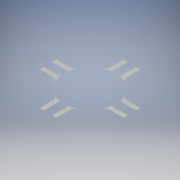
# Autodesk Inventor part: center
Saved by Autodesk Inventor 2016 (Build 200138000, 138)
## iProperties
Created: 2016-02-28
Part Number: center
Material: Generic
Document SubType Name: Modeling
Designer: Matt Ruffner
Density: 1 g/cm^3
Appearance: Default
Author: Matt Ruffner
Autodesk Inventor part; units mm, degrees
ref_plane "YZ Plane" through (0, 0, 0) normal (1, 0, 0) x (0, 1, 0)
ref_plane "XZ Plane" through (0, 0, 0) normal (0, 1, 0) x (-1, 0, 0)
ref_plane "XY Plane" through (0, 0, 0) normal (0, 0, 1) x (1, 0, 0)
sketch "Sketch1" plane through (0, 0, 0) normal (0, 1, 0) x (-1, 0, 0)
  circle A0 centre (0, 0) radius 4.318
  line L0 (0, -31.496) -> (5.08, -31.496)
  line L1 (0, -31.496) -> (-5.08, -31.496)
  line L2 (31.496, 0) -> (31.496, 5.08)
  line L3 (31.496, 0) -> (31.496, -5.08)
  line L4 (0, 31.496) -> (-5.08, 31.496)
  line L5 (0, 31.496) -> (5.08, 31.496)
  line L6 (-31.496, 0) -> (-31.496, -5.08)
  line L7 (-31.496, 0) -> (-31.496, 5.08)
  line L8 (31.496, 5.08) -> (50.5454, 5.08)
  line L9 (31.496, -5.08) -> (50.5454, -5.08)
  line L10 (5.08, -31.496) -> (5.08, -50.5454)
  line L11 (-5.08, -31.496) -> (-5.08, -50.5454)
  line L12 (-31.496, -5.08) -> (-50.5454, -5.08)
  line L13 (-31.496, 5.08) -> (-50.5454, 5.08)
  line L14 (-5.08, 31.496) -> (-5.08, 50.5454)
  line L15 (5.08, 31.496) -> (5.08, 50.5454)
  line L16 (-50.5454, 5.08) -> (-50.5454, 10.16)
  line L17 (-50.5454, -5.08) -> (-50.5454, -10.16)
  line L18 (-5.08, -50.5454) -> (-10.16, -50.5454)
  line L19 (5.08, -50.5454) -> (10.16, -50.5454)
  line L20 (50.5454, -5.08) -> (50.5454, -10.16)
  line L21 (50.5454, 5.08) -> (50.5454, 10.16)
  line L22 (5.08, 50.5454) -> (10.16, 50.5454)
  line L23 (-5.08, 50.5454) -> (-10.16, 50.5454)
  line L24 (-10.16, 50.5454) -> (-10.16, 29.8123)
  line L25 (10.16, 50.5454) -> (10.16, 29.8123)
  line L26 (-50.5454, 10.16) -> (-29.8123, 10.16)
  line L27 (-50.5454, -10.16) -> (-29.8123, -10.16)
  line L28 (-10.16, -50.5454) -> (-10.16, -29.8123)
  line L29 (10.16, -50.5454) -> (10.16, -29.8123)
  line L30 (50.5454, -10.16) -> (29.8123, -10.16)
  line L31 (50.5454, 10.16) -> (29.8123, 10.16)
  arc A1 (-10.16, 29.8123) -> (-29.8123, 10.16) centre (0, 0) ccw
  arc A2 (-29.8123, -10.16) -> (-10.16, -29.8123) centre (0, 0) ccw
  arc A3 (10.16, -29.8123) -> (29.8123, -10.16) centre (0, 0) ccw
  arc A4 (29.8123, 10.16) -> (10.16, 29.8123) centre (0, 0) ccw
  dimension "d7" = 360
  dimension "d13" = 360
  dimension "d0" = 8.636
  dimension "d9" = 5.08
  dimension "d10" = 5.08
  constraints: 64 end point, 8 horizontal, 8 point on circle, 5 centre point, 4 parallel, 4 vertical, 3 perpendicular, 1 coincident, 1 point on line, 46 other
  measures "d0" diameter of A0
  measures "d9" distance of L13.end L16.end
  measures "d10" distance of L12.end L17.end
extrude "Extrusion1" add sketch "Sketch1" along normal blind 7.62
sketch "Sketch2" plane through (10.16, 0, 50.5454) normal (1, 0, 0) x (0, 0, -1)
  line L0 (0, 0) -> (20.7331, 0) projected
  circle A0 centre (11.1754, 3.81) radius 1.651
  point P0 (50.5454, 0)
  dimension "d19" = 3.302
  constraints: 1 centre point
  measures "d19" diameter of A0
extrude "Extrusion2" cut sketch "Sketch2" against normal up to surface (20.32 mm away)
pattern_circular "Circular Pattern1" count 4 over 360 about axis through (0, 0, 0) along (0, 1, 0) of "Extrusion2"
sketch "Sketch3" plane through (0, 7.62, 0) normal (0, 1, 0) x (1, 0, 0)
  circle A0 centre (0, 0) radius 31.369
  circle A1 centre (0, 0) radius 11.2522
  dimension "d25" = 62.738
  dimension "d26" = 22.5044
  constraints: 2 centre point, 2 coincident
  measures "d25" diameter of A0
  measures "d26" diameter of A1
extrude "Extrusion3" add sketch "Sketch3" along normal blind 4.826
sketch "Sketch4" plane through (0, 7.62, 0) normal (0, 1, 0) x (1, 0, 0)
  circle A0 centre (0, 0) radius 11.2522 projected
extrude "Extrusion4" cut sketch "Sketch4" against normal blind 2.54
chamfer "Chamfer1" distance 3.175 angle 45 8 edges at (10.16, 3.81, 29.8123) (29.8123, 3.81, 10.16) (-10.16, 3.81, 29.8123) (-29.8123, 3.81, 10.16) (-29.8123, 3.81, -10.16) (-10.16, 3.81, -29.8123) (10.16, 3.81, -29.8123) (29.8123, 3.81, -10.16)
body "Solid1"
